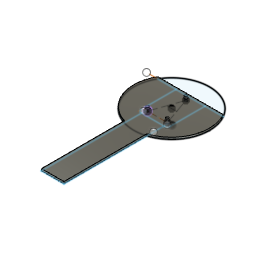
Roboter-Platte-v1 (Autodesk Fusion 360 design; units mm, degrees)
Autodesk Fusion 360 part; units mm, degrees
note: some values were not read from the file. Set by a fixed rule: which sketch regions a step uses.
sketch "Skizze1" plane through (0, 0, 0) normal (0, 0, 1) x (1, 0, 0)
sketch "Skizze2" plane through (0, 0, 0) normal (0, 0, 1) x (1, 0, 0)
  circle A0 centre (0, 0) radius 1.4
  circle A1 centre (21, 0) radius 1.4
  circle A2 centre (10.5, 30.2) radius 1.4
  line L0 (22.4, 0) -> (22.4, -16) construction
  line L1 (-1.4, 0) -> (22.4, 0) construction
  line L2 (22.4, 0) -> (22.4, -111)
  line L3 (22.4, -111) -> (-1.4, -111)
  line L4 (-1.4, -111) -> (-1.4, 0)
  line L5 (-1.4, 0) -> (-4.9, 0) construction
  line L6 (22.4, 0) -> (25.9, 0) construction
  line L7 (-4.9, 0) -> (-4.9, -5) construction
  line L8 (-1.9, -5) -> (22.9, -5)
  line L9 (25.9, -2) -> (25.9, 35)
  line L10 (25.9, 35) -> (-4.9, 35)
  line L11 (-4.9, 35) -> (-4.9, -2)
  arc A3 (22.9, -5) -> (25.9, -2) centre (22.9, -2) ccw
  arc A4 (-4.9, -2) -> (-1.9, -5) centre (-1.9, -2) ccw
  line L12 (10.5, 30.2) -> (0, 0) construction
  line L13 (21, 0) -> (10.5, 30.2) construction
  line L14 (0, 0) -> (21, 0) construction
  line L15 (15.75, 15.1) -> (5.25, 15.1) construction
  circle A5 centre (10.5, 15.1) radius 40
  line L16 (-4.9, 35) -> (-24.1986, 35)
  line L17 (-24.1986, 35) -> (-36, 35) construction
  line L18 (25.9, 35) -> (45.1986, 35)
  dimension "d1" = 2.8
  dimension "d2" = 2.8
  dimension "d3" = 21
  dimension "d5" = 2.8
  dimension "d6" = 30.2
  dimension "d7" = 10.5
  dimension "d24" = 111
  dimension "d25" = 3.5
  dimension "d26" = 3.5
  dimension "d27" = 40
  dimension "d28" = 3
  dimension "d29" = 3
  dimension "d30" = 80
  constraint coincident A0.centre L12.end
  constraint coincident A1 L0.start
  constraint tangent A1 L0
  constraint vertical L0
  constraint horizontal L1
  constraint vertical L2
  constraint horizontal L3
  constraint vertical L4
  constraint coincident A0 L1.start
  constraint perpendicular L4 L5
  constraint perpendicular L2 L6
  constraint perpendicular L5 L7
  constraint horizontal L8
  constraint vertical L9
  constraint horizontal L10
  constraint vertical L11
  constraint tangent L8 A3
  constraint tangent L9 A3
  constraint coincident L7.end L8
  constraint coincident L7.end L11
  constraint tangent L8 A4
  constraint tangent L11 A4
  constraint coincident A2.centre L12.start
  constraint coincident A1.centre L13.start
  constraint parallel L1 L14
  constraint midpoint L13 L15.start
  constraint midpoint L12 L15.end
  constraint midpoint L15 A5.centre
  constraint coincident A5 L16.end
  constraint perpendicular L11 L16
  constraint parallel L16 L17
  constraint coincident A5 L18.end
  constraint perpendicular L9 L18
  measures "d1" diameter of A0
  measures "d2" diameter of A1
  measures "d3" distance of A1.centre A0.centre
  measures "d5" diameter of A2
  measures "d6" vertical distance of A0.centre A2.centre
  measures "d7" horizontal distance of A0.centre A2.centre
  measures "d24" distance of L1.start L3.end
  measures "d25" distance of L1.start L5.end
  measures "d26" distance of L0.start L6.end
  measures "d27" distance of L7.end L10.end
  measures "d28" radius of A3
  measures "d29" radius of A4
  measures "d30" diameter of A5
extrude "Extrusion1" add sketch "Skizze2" along normal blind 2 contours L8 L9 L10 L11 A3 A4
extrude "Extrusion2" add sketch "Skizze2" along normal blind 4.25 contours A2
extrude "Extrusion3" add sketch "Skizze2" along normal blind 4.25 contours A0 | A1
fillet "Abrundung1" [no effect]
fillet "Abrundung2" [no effect]
fillet "Abrundung3" [no effect]
fillet "Abrundung4" [no effect]
fillet "Abrundung5" [no effect]
extrude "Extrusion4" add sketch "Skizze2" along normal blind 2 contours L2 L8 L9 A3 A5 L18 | L2 L4 L8 A5 | L4 L8 L11 A4 A5 L16
extrude "Extrusion5" add sketch "Skizze2" along normal blind 2 contours L2 L3 L4 A5
equation "d3 = 23.8 mm - 2.8 mm"
equation "d6 = 33 mm - 2.8 mm"
equation "d7 = ( 21 / 2 ) * 1 mm"
